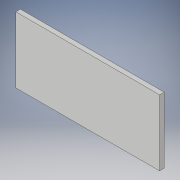
# Autodesk Inventor part: pcb
Saved by Autodesk Inventor 2017 (Build 210142000, 142)
## iProperties
Created: 2017-04-10
Part Number: pcb
Material: Generic
Document SubType Name: Modeling
Designer: Adrian Negrean2
Density: 1 g/cm^3
Appearance: Default
Author: Adrian Negrean2
Autodesk Inventor part; units mm, degrees
ref_plane "YZ Plane" through (0, 0, 0) normal (1, 0, 0) x (0, 1, 0)
ref_plane "XZ Plane" through (0, 0, 0) normal (0, 1, 0) x (-1, 0, 0)
ref_plane "XY Plane" through (0, 0, 0) normal (0, 0, 1) x (1, 0, 0)
sketch "Sketch1" plane through (0, 0, 0) normal (0, 0, 1) x (1, 0, 0)
  line L0 (-19.0113, 11.8059) -> (30.7887, 11.8059)
  line L1 (30.7887, 11.8059) -> (30.7887, -10.9941)
  line L2 (30.7887, -10.9941) -> (-19.0113, -10.9941)
  line L3 (-19.0113, -10.9941) -> (-19.0113, 11.8059)
  point P0 (0, 0)
  dimension "d0" = 22.8
  dimension "d1" = 49.8
  constraints: 8 end point, 2 parallel, 1 horizontal, 1 perpendicular
  measures "d0" distance of L2.end L0.start
  measures "d1" distance of L1.end L2.end
extrude "Extrusion1" add sketch "Sketch1" along normal blind 1.6
body "Solid1"
